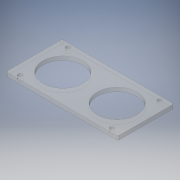
# Autodesk Inventor part: EndStück_Caps
Saved by Autodesk Inventor 2016 (Build 200138000, 138)
## iProperties
Created: 2018-05-15
Part Number: EndStück_Caps
Material: Polycarbonate, Clear
Document SubType Name: Modeling
Designer: Phil Erle
Density: 1.2 g/cm^3
Appearance: Polycarbonate - Clear
Author: Phil Erle
Autodesk Inventor part; units mm, degrees
ref_plane "YZ Plane" through (0, 0, 0) normal (1, 0, 0) x (0, 1, 0)
ref_plane "XZ Plane" through (0, 0, 0) normal (0, 1, 0) x (-1, 0, 0)
ref_plane "XY Plane" through (0, 0, 0) normal (0, 0, 1) x (1, 0, 0)
sketch "Sketch1" plane through (0, 0, 0) normal (0, 0, 1) x (1, 0, 0)
  line L0 (-70, -35) -> (70, -35)
  line L1 (70, -35) -> (70, 35)
  line L2 (70, 35) -> (-70, 35)
  line L3 (-70, 35) -> (-70, -35)
  line L4 (-70, -35) -> (70, 35) construction
  line L5 (70, -35) -> (-70, 35) construction
  point P0 (0, 0)
  dimension "d0" = 140
  dimension "d1" = 70
  constraints: 12 end point, 2 midpoint, 2 parallel, 1 horizontal, 1 perpendicular
  measures "d0" distance of L1.end L2.end
  measures "d1" distance of L0.end L1.end
extrude "Extrusion1" add sketch "Sketch1" along normal blind 5
sketch "Sketch2" plane through (0, 0, 5) normal (0, 0, 1) x (1, 0, 0)
  line L0 (-57.5, -30) -> (57.5, -30) construction
  line L1 (57.5, -30) -> (57.5, 30) construction
  line L2 (57.5, 30) -> (-57.5, 30) construction
  line L3 (-57.5, 30) -> (-57.5, -30) construction
  line L4 (-57.5, -30) -> (57.5, 30) construction
  line L5 (57.5, -30) -> (-57.5, 30) construction
  point P0 (0, 0)
  dimension "d4" = 115
  dimension "d5" = 60
  constraints: 12 end point, 4 coincident, 2 midpoint, 2 parallel, 1 horizontal, 1 perpendicular
  measures "d4" distance of L2.end L1.end
  measures "d5" distance of L1.end L0.end
hole "Hole1" at (-57.5, -30, 5) at (-57.5, 30, 5) at (57.5, 30, 5) at (57.5, -30, 5) direction (0, 0, -1) diameter 5.5 depth 8 tip angle 118 clearance for "Countersunk Flat Head Screw DIN EN ISO 2009" size "M5" standard "DIN"
fillet "Fillet1" radius 2 4 edges at (70, 35, 2.5) (70, -35, 2.5) (-70, 35, 2.5) (-70, -35, 2.5)
sketch "Sketch3" plane through (0, 0, 5) normal (0, 0, 1) x (1, 0, 0)
  circle A0 centre (-34, 0) radius 25
  circle A1 centre (34, 0) radius 25
  line L0 (-34, 0) -> (34, 0) construction
  point P0 (0, 0)
  point P1 (0, 0)
  dimension "d14" = 50
  dimension "d15" = 50
  dimension "d16" = 68
  constraints: 2 centre point, 2 end point, 1 coincident, 1 horizontal, 1 midpoint
  measures "d14" diameter of A0
  measures "d15" diameter of A1
  measures "d16" distance of L0.end L0.start
extrude "Extrusion2" cut sketch "Sketch3" against normal blind 5
body "Solid1"
